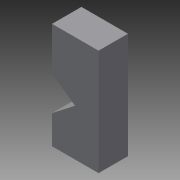
# Autodesk Inventor part: Notch_example
Saved by Autodesk Inventor 2015 (Build 190159000, 159)
## iProperties
Created: 2015-01-30
Part Number: Notch_example
Material: Generic
Document SubType Name: Modeling
Designer: admin
Density: 1 g/cm^3
Appearance: Default
Author: admin
Autodesk Inventor part; units mm, degrees
ref_plane "YZ Plane" through (0, 0, 0) normal (1, 0, 0) x (0, 1, 0)
ref_plane "XZ Plane" through (0, 0, 0) normal (0, 1, 0) x (-1, 0, 0)
ref_plane "XY Plane" through (0, 0, 0) normal (0, 0, 1) x (1, 0, 0)
sketch "Sketch1" plane through (0, 0, 0) normal (0, 1, 0) x (-1, 0, 0)
  line L0 (-4.019, -7.9168) -> (3.8978, -7.9168)
  line L1 (3.8978, -7.9168) -> (3.8978, 10.1384)
  line L2 (3.8978, 10.1384) -> (-4.019, 10.1384)
  line L3 (-4.019, 10.1384) -> (-4.019, -7.9168)
  point P0 (0, 0)
  constraints: 8 end point, 2 parallel, 1 horizontal, 1 perpendicular
extrude "Extrusion1" add sketch "Sketch1" along normal blind 5
sketch "Sketch2" plane through (0, 5, 0) normal (0, 1, 0) x (1, 0, 0)
  line L0 (-3.8978, -2.87) -> (0, 0)
  line L1 (0, 0) -> (-3.8978, 3.0252)
  line L2 (4.019, 7.9168) -> (-3.8978, 7.9168) projected
  line L3 (-3.8978, 7.9168) -> (-3.8978, -10.1384) projected
  line L4 (-3.8978, -10.1384) -> (4.019, -10.1384) projected
  line L5 (4.019, -10.1384) -> (4.019, 7.9168) projected
  constraints: 4 end point, 2 point on line
extrude "Extrusion2" cut sketch "Sketch2" against normal blind 5 contours L3 L1 L0
body "Solid1"
